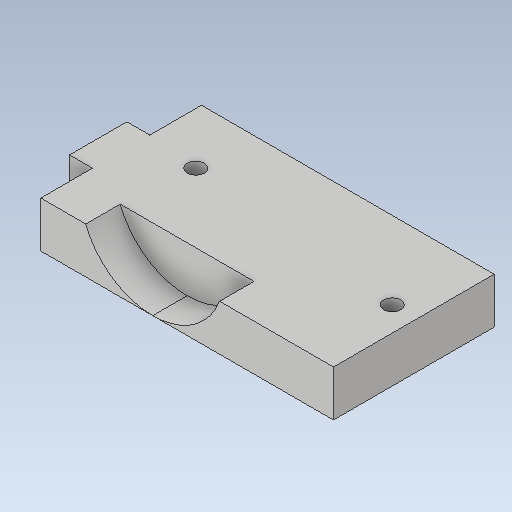
# Autodesk Inventor part: arm_2_microservo_case
Saved by Autodesk Inventor 2020.1 (Build 241239000, 239)
## iProperties
Created: 2018-02-08
Part Number: arm_2_microservo_case
Material: Genérico
Document SubType Name: Modeling
Designer: se_ma
Density: 1 g/cm^3
Appearance: Valor por defecto
Author: se_ma
Autodesk Inventor part; units mm, degrees
ref_plane "YZ Plane" through (0, 0, 0) normal (1, 0, 0) x (0, 1, 0)
ref_plane "XZ Plane" through (0, 0, 0) normal (0, 1, 0) x (-1, 0, 0)
ref_plane "XY Plane" through (0, 0, 0) normal (0, 0, 1) x (1, 0, 0)
sketch "Boceto1" plane through (0, 0, 0) normal (0, 1, 0) x (-1, 0, 0)
  line L0 (0, 0) -> (51, 0)
  line L1 (51, 0) -> (51, -28)
  line L2 (51, -28) -> (0, -28)
  line L3 (0, -28) -> (0, 0)
  line L4 (51, 0) -> (51, -18.5)
  line L5 (51, -18.5) -> (42, -18.5)
  circle A0 centre (42, -18.5) radius 1.5
  line L6 (0, 0) -> (0, -14.5)
  line L7 (0, -14.5) -> (4.25, -14.5)
  circle A1 centre (4.25, -14.5) radius 1.5
  line L8 (51, 0) -> (51, -14)
  line L9 (51, -14) -> (55, -14)
  line L10 (55, -14) -> (55, -9)
  line L11 (55, -9) -> (51, -9)
  line L12 (55, -14) -> (55, -19)
  line L13 (55, -19) -> (51, -19)
  dimension "d0" = 51
  dimension "d1" = 28
  dimension "d2" = 18.5
  dimension "d3" = 9
  dimension "d4" = 3
  dimension "d5" = 14.5
  dimension "d6" = 4.25
  dimension "d7" = 3
  dimension "d8" = 14
  dimension "d9" = 4
  dimension "d10" = 5
  dimension "d11" = 5
  constraints: 28 end point, 7 perpendicular, 6 point on line, 2 centre point, 2 coincident, 2 parallel, 1 horizontal
  measures "d0" distance of L1.end L2.end
  measures "d1" distance of L0.end L1.end
  measures "d2" distance of L0.end L4.end
  measures "d3" distance of L4.end L5.end
  measures "d4" diameter of A0
  measures "d5" distance of L0.start L6.end
  measures "d6" distance of L6.end L7.end
  measures "d7" diameter of A1
  measures "d8" distance of L0.end L8.end
  measures "d9" distance of L8.end L9.end
  measures "d10" distance of L9.end L10.end
  measures "d11" distance of L9.end L12.end
extrude "Extrusión1" add sketch "Boceto1" along normal blind 2
sketch "Boceto2" plane through (0, 0, 0) normal (0, -1, 0) x (1, 0, 0)
  circle A0 centre (-42, -18.5) radius 1.5 projected
  circle A1 centre (-42, -18.5) radius 1.5
  point P0 (0, 0)
  constraints: 1 centre point, 1 coincident
extrude "Extrusión2" add sketch "Boceto2" against normal blind 2
sketch "Boceto3" plane through (0, 0, 0) normal (0, -1, 0) x (1, 0, 0)
  circle A0 centre (-4.25, -14.5) radius 1.5 projected
  circle A1 centre (-4.25, -14.5) radius 1.5
  line L0 (-51, 0) -> (0, 0) projected
  line L1 (0, 0) -> (-51, 0)
  line L2 (-51, -9) -> (-51, 0) projected
  line L3 (-51, 0) -> (-51, -9)
  line L4 (-55, -9) -> (-51, -9) projected
  line L5 (-51, -9) -> (-55, -9)
  line L6 (-51, -19) -> (-55, -19) projected
  line L7 (-55, -9) -> (-55, -19)
  line L8 (-55, -19) -> (-51, -19)
  line L9 (-51, -28) -> (-51, -19) projected
  line L10 (-51, -19) -> (-51, -28)
  line L11 (0, -28) -> (-51, -28) projected
  line L12 (-51, -28) -> (0, -28)
  line L13 (0, 0) -> (0, -28) projected
  line L14 (0, -28) -> (0, 0)
  constraints: 16 end point, 4 collinear, 4 perpendicular, 1 centre point, 1 coincident
extrude "Extrusión3" add sketch "Boceto3" along normal blind 6
sketch "Boceto4" plane through (0, -6, 0) normal (0, -1, 0) x (1, 0, 0)
  line L0 (-51, 0) -> (-51, -9) projected
  line L1 (-51, -9) -> (-51, -18)
  line L2 (-51, -18) -> (-42, -18)
  circle A0 centre (-42, -18) radius 1.5
  point P0 (0, 0)
  dimension "d18" = 9
  dimension "d19" = 9
  dimension "d20" = 3
  constraints: 4 end point, 1 centre point, 1 coincident, 1 perpendicular, 1 vertical
  measures "d18" distance of L0.end L1.end
  measures "d19" distance of L1.end L2.end
  measures "d20" diameter of A0
extrude "Extrusión4" cut sketch "Boceto4" against normal blind 8
sketch "Boceto5" plane through (-51, 2, 0) normal (0, 0, 1) x (1, 0, 0)
  line L0 (51, -8) -> (51, 17)
  line L1 (-4, 4.5) -> (19.5, 4.5)
  circle A0 centre (19.5, 4.5) radius 12.5
  line L2 (0, -8) -> (51, -8) projected
  line L3 (51, 0) -> (0, 0) projected
  line L4 (7.8381, 0) -> (31.1619, 0)
  point P0 (51, -2)
  dimension "d23" = 25
  dimension "d24" = 23.5
  constraints: 6 end point, 2 point on circle, 2 point on line, 1 centre point, 1 coincident, 1 tangent, 1 vertical
  measures "d23" distance of L0.start L0.end
  measures "d24" distance of L1.start L1.end
extrude "Extrusión5" cut sketch "Boceto5" against normal blind 6 contours A0 L3 picked at (19.5, -2.6667)
